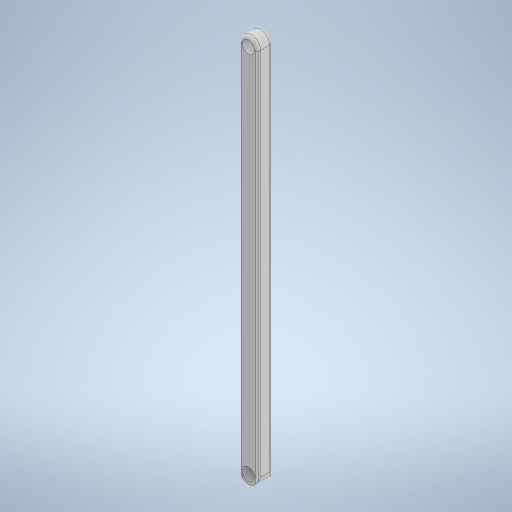
# Autodesk Inventor part: Metallstange
Saved by Autodesk Inventor 2023 (Build 270158000, 158)
## iProperties
Created: 2024-02-03
Part Number: Metallstange
Material: Generisch
Document SubType Name: Modeling
Designer: jefar
Density: 1 g/cm^3
Appearance: Vorgabe
Author: jefar
Autodesk Inventor part; units mm, degrees
ref_plane "YZ Plane" through (0, 0, 0) normal (1, 0, 0) x (0, 1, 0)
ref_plane "XZ Plane" through (0, 0, 0) normal (0, 1, 0) x (-1, 0, 0)
ref_plane "XY Plane" through (0, 0, 0) normal (0, 0, 1) x (1, 0, 0)
sketch "Skizze1" plane through (0, 0, 0) normal (0, 0, 1) x (1, 0, 0)
  line L0 (-210, 0) -> (210, 0) construction
  line L1 (0, -150) -> (0, 200) construction
  arc A0 (150, 0) -> (-150, 0) centre (0, 0) ccw
  line L2 (-150, 0) -> (150, 0)
  circle A1 centre (0, 0) radius 100
  dimension "d14" = 200
  constraints: 2 centre point, 2 coincident, 2 end point, 2 point on circle, 2 point on line
  measures "d14" diameter of A1
sketch "Skizze2" plane through (0, 0, 0) normal (0, 0, 1) x (1, 0, 0)
  point P0 (0, 0)
extrude "Extrusion1" add sketch "Skizze1" along normal blind 250 contours L2 A1 A0 | L2 A1 picked at (21.5157, 33.3544)
fillet "Rundung1" radius 50 2 edges at (0, 150, 250) (0, 150, 0)
sketch "Skizze3" plane through (-100, 0, 0) normal (0, -1, 0) x (1, 0, 0)
  circle A0 centre (100, 125) radius 175
  point P0 (100, 0)
  dimension "d4" = 350
  constraints: 1 centre point
  measures "d4" diameter of A0
extrude "Extrusion2" add sketch "Skizze3" along normal blind 6100
fillet "Rundung2" [suppressed]
sketch "Skizze4" plane through (-100, 0, 0) normal (0, 1, 0) x (1, 0, 0)
  circle A0 centre (100, -125) radius 175 projected
  arc A1 (-22.4745, 0) -> (100, 50) centre (100, -125) ccw
  arc A2 (222.4745, 0) -> (-22.4745, 0) centre (100, -125) ccw
  line L0 (-22.4745, 0) -> (222.4745, 0)
  line L1 (0, 0) -> (200, 0) projected
  arc A3 (-22.4745, -250) -> (222.4745, -250) centre (100, -125) ccw
  line L2 (-22.4745, -250) -> (222.4745, -250)
  line L3 (200, -250) -> (0, -250) projected
  point P0 (100, 0)
  point P1 (-22.4745, -250)
  constraints: 12 point on circle, 4 end point, 3 centre point, 3 concentric, 2 collinear
extrude "Extrusion3" cut sketch "Skizze4" against normal blind 6100 contours L0 A0
extrude "Extrusion4" cut sketch "Skizze4" against normal blind 6100 contours A0 L2
sketch "Skizze5" plane through (-100, 0, 0) normal (0, 1, 0) x (1, 0, 0)
  arc A0 (240, -230) -> (240, -20) centre (100, -125) ccw projected
  arc A1 (250, -50) -> (240, -20) centre (200, -50) ccw projected
  arc A2 (240, -230) -> (240, -20) centre (100, -125) ccw
  line L0 (250, -50) -> (-50, -50) projected
  arc A3 (240, -230) -> (250, -200) centre (200, -200) ccw projected
  line L1 (250, -50) -> (250, -200)
  line L2 (250, -50) -> (250, -200) projected
  arc A4 (240, -230) -> (250, -200) centre (200, -200) ccw
  line L3 (100, 0) -> (100, -250)
  line L4 (200, -250) -> (0, -250) projected
  arc A5 (0, 0) -> (-40, -20) centre (0, -50) ccw projected
  arc A6 (-40, -20) -> (-40, -230) centre (100, -125) ccw projected
  arc A7 (-40, -20) -> (-40, -230) centre (100, -125) ccw
  line L5 (-50, -200) -> (250, -200) projected
  line L6 (-50, -50) -> (-50, -200)
  arc A8 (-40, -20) -> (-50, -50) centre (0, -50) ccw projected
  arc A9 (-40, -20) -> (-50, -50) centre (0, -50) ccw
  line L7 (-50, -50) -> (-50, -200) projected
  arc A10 (-50, -200) -> (-40, -230) centre (0, -200) ccw projected
  arc A11 (-50, -200) -> (-40, -230) centre (0, -200) ccw
  constraints: 10 point on circle, 6 end point, 5 centre point, 1 midpoint, 1 tangent, 1 vertical
extrude "Extrusion5" cut sketch "Skizze5" against normal blind 6100 contours A3 L1 A1 A0 | A10 A6 A8 L6
extrude "Extrusion6" cut sketch "Skizze1" along normal blind 6100 contours A1 L2 | L2 A1
sketch "Skizze6" plane through (0, 0, 250) normal (0, 0, 1) x (1, 0, 0)
  circle A0 centre (0, -6100) radius 150
  circle A1 centre (0, -6100) radius 100
  line L0 (150, -6100) -> (-150, -6100)
  line L1 (-122.4745, -6100) -> (122.4745, -6100) projected
  line L2 (201.0424, -6100) -> (-326.8055, -6100)
  circle A2 centre (0, -6100) radius 100
  point P0 (0, 0)
  point P1 (-100, -6100)
  point P2 (100, -6100)
  dimension "d17" = 300
  dimension "d18" = 200
  constraints: 4 end point, 3 centre point, 2 coincident, 2 point on circle, 1 collinear, 1 concentric, 1 point on line
  measures "d17" diameter of A0
  measures "d18" diameter of A1
extrude "Extrusion7" add sketch "Skizze6" against normal blind 250 contours A0 L0 A1 picked at (-121.6685, -6120.1193)
sketch "Skizze7" plane through (-150, -6100, 250) normal (0, 1, 0) x (1, 0, 0)
  line L0 (27.5255, 0) -> (50, 0) projected
  line L1 (27.5255, 0) -> (0, 0) projected
  line L2 (27.5255, 0) -> (0, 0)
  line L3 (0, 0) -> (0, 50) projected
  line L4 (0, 0) -> (0, 50)
  arc A0 (0, 50) -> (10, 20) centre (50, 50) ccw projected
  arc A1 (10, 20) -> (50, 0) centre (50, 50) ccw projected
  arc A2 (0, 50) -> (50, 0) centre (50, 50) ccw
  line L5 (250, 0) -> (50, 0) projected
  line L6 (27.5255, 0) -> (50, 0)
  point P0 (150, 250)
  constraints: 6 end point, 3 collinear, 3 point on circle, 1 centre point, 1 concentric, 1 point on line
extrude "Extrusion8" cut sketch "Skizze7" against normal blind 250
sketch "Skizze8" plane through (122.4745, -6100, 250) normal (0, 1, 0) x (1, 0, 0)
  arc A0 (0, 0) -> (17.5255, 20) centre (-122.4745, 125) ccw projected
  line L0 (27.5255, 0) -> (0, 0) projected
  line L1 (0, 0) -> (27.5255, 0)
  line L2 (27.5255, 0) -> (27.5255, 50) projected
  line L3 (27.5255, 0) -> (27.5255, 50)
  arc A1 (-22.4745, 0) -> (17.5255, 20) centre (-22.4745, 50) ccw projected
  arc A2 (-22.4745, 0) -> (27.5255, 50) centre (-22.4745, 50) ccw
  line L4 (27.5255, 200) -> (27.5255, 250) projected
  line L5 (27.5255, 200) -> (27.5255, 250)
  line L6 (27.5255, 250) -> (-19.2004, 250)
  line L7 (27.5255, 250) -> (-272.4745, 250) projected
  line L8 (27.5255, 200) -> (27.5255, 50) projected
  arc A3 (27.5255, 200) -> (-19.2004, 250) centre (-22.5892, 200) ccw
  line L9 (-272.4745, 200) -> (-272.4745, 250) projected
  line L10 (-272.4745, 200) -> (-272.4745, 250)
  arc A4 (-262.4745, 230) -> (-272.4745, 200) centre (-222.4745, 200) ccw projected
  arc A5 (-222.4745, 250) -> (-262.4745, 230) centre (-222.4745, 200) ccw projected
  line L11 (-272.4745, 250) -> (-222.4745, 250)
  arc A6 (-222.4745, 250) -> (-272.4745, 200) centre (-222.4745, 200) ccw
  line L12 (27.5255, 200) -> (27.5255, 250)
  point P0 (-122.4745, 250)
  point P1 (17.5255, 20)
  constraints: 14 end point, 6 point on circle, 6 tangent, 5 collinear, 3 centre point, 1 perpendicular, 1 point on line
extrude "Extrusion9" cut sketch "Skizze8" against normal blind 250
extrude "Extrusion10" cut sketch "Skizze6" against normal through all contours L0 A1 picked at (-30.5737, -6077.6422)
